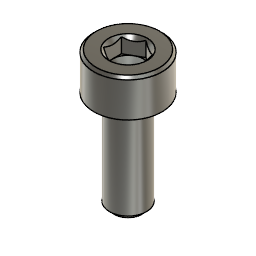
M3 Parametric SHCS (Autodesk Fusion 360 design; units mm, degrees)
part number: M3x8mm SHCS
Autodesk Fusion 360 part; units mm, degrees
sketch "Sketch2" plane through (0, 0, 0) normal (1, 0, 0) x (0, 1, 0)
  line L0 (-1.5, -10.6) -> (-1.1, -11)
  line L1 (2.75, 0) -> (-2.75, 0)
  line L2 (-2.75, -0.2) -> (-2.75, -3)
  line L3 (-1.1, -11) -> (0, -11)
  line L4 (0, -2.0511) -> (0, -3)
  line L5 (-1.25, -0.3) -> (-1.55, 0)
  line L6 (-2.75, -3) -> (-1.5, -3)
  line L7 (-1.25, -1.3) -> (-1.25, -0.3)
  line L8 (-1.25, -1.3) -> (0, -2.0511)
  line L9 (-2.55, 0) -> (-2.75, -0.2)
  line L10 (0, 0) -> (0, -2.0511)
  line L11 (0, -11) -> (0, -3)
  line L12 (-1.5, -3) -> (-1.5, -10.6)
  point P0 (-1.75, 2)
  point P1 (0, -3)
  dimension "d16" = 1.25
  dimension "d19" = 3
  dimension "d20" = 1.3
  dimension "d21" = 59
  dimension "d22" = 5.5
  dimension "d23" = 45
  dimension "d24" = 1.5
  dimension "d25" = 45
  dimension "d26" = 0.4
  dimension "d27" = 8
  dimension "d28" = 0.2
  dimension "d34" = 0.3
  dimension "d35" = 45
  constraint coincident L10.start L1
  constraint perpendicular L1 L10
  constraint midpoint L10.start L1
  constraint perpendicular L1 L7
  constraint coincident L4.start L10
  constraint coincident L4.start L8.end
  constraint coincident L5.end L1
  constraint coincident P1 L10
  constraint coincident L9.start L1
  constraint coincident L1.end L2
  constraint perpendicular L2 L6
  constraint perpendicular L6 L12
  constraint perpendicular L3 L12
  constraint coincident P1 L4.end
  constraint coincident P1 L6
  constraint parallel L2 L4
  constraint horizontal L1
  measures "d16" distance of L7 L10
  measures "d19" distance of P1 L1
  measures "d20" distance of L7.start L1
  measures "d21" angle of L8 L10
  measures "d22" distance of L1.end L1.start
  measures "d23" angle of L1 L9
  measures "d24" distance of L11 L12
  measures "d25" angle of L0 L12
  measures "d26" distance of L0.end L12
  measures "d27" distance of L3 L6
  measures "d28" distance of L9.start L1.end
  measures "d34" horizontal distance of L5.end L5.start
  measures "d35" angle of L5 L7
revolve "Revolve1" add sketch "Sketch2" angle 360 about axis through (0, 0, 0) along (0, 0, -1) contours L0 L1 L2 L3 L4 L5 L6 L7 L8 L9 L11 L12
sketch "Sketch3" plane through (0, 0, 0) normal (0, 0, 1) x (1, 0, 0)
  line L0 (1.25, 0.7217) -> (0, 1.4434)
  line L1 (0, 1.4434) -> (-1.25, 0.7217)
  line L2 (-1.25, 0.7217) -> (-1.25, -0.7217)
  line L3 (-1.25, -0.7217) -> (0, -1.4434)
  line L4 (0, -1.4434) -> (1.25, -0.7217)
  line L5 (1.25, -0.7217) -> (1.25, 0.7217)
  dimension "d31" = 1.25
  constraint vertical L5
  measures "d31" distance of origin L5
extrude "Extrude4" cut sketch "Sketch3" against normal up to surface (1.3 mm away)
equation "Length = 8 mm"
equation "d16 = ( 2.5 / 2 ) * 1 mm"
equation "d26 = 0.5 mm * 0.8"
equation "d27 = Length"
equation "d31 = ( 2.5 / 2 ) * 1 mm"
